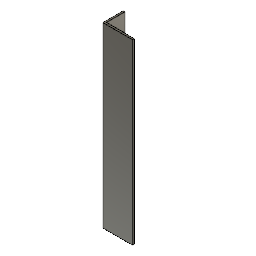
angle_bracket (Autodesk Fusion 360 design; units mm, degrees)
Autodesk Fusion 360 part; units mm, degrees
box "PrimitivaParallelepipedo1" add length 2 width 15 height 95 placed x (0, 1, 0) y (-1, 0, 0) z (0, 0, 1) at (15, 0, 0)
extrude "Estrusione1" add 1 faces at (15, 0.6667, 31.6667) along direction (1, 0, 0) blind 2
box "PrimitivaParallelepipedo2" add length 10 width 2 height 95 placed x (0, 1, 0) y (-1, 0, 0) z (0, 0, 1) at (2, 0, 0)
extrude "Estrusione2" add 1 faces at (1.3333, 10, 31.6667) along direction (0, 1, 0) blind 2
move_face "FacceDiOffset1" offset -1 1 faces at (5.6667, 0, 31.6667)
move_face "FacceDiOffset2" offset -1 1 faces at (0, 4.6667, 31.6667)
